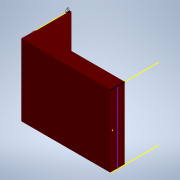
# Autodesk Inventor part: LPS_base
Saved by Autodesk Inventor 2022 (Build 260153000, 153)
## iProperties
Created: 2024-07-06
Part Number: LPS_base
Material: Типовые
Document SubType Name: Modeling
Designer: Капустяник Андрей
Density: 1 g/cm^3
Appearance: По умолчанию
Author: Капустяник Андрей
Autodesk Inventor part; units mm, degrees
ref_plane "YZ Plane" through (0, 0, 0) normal (1, 0, 0) x (0, 1, 0)
ref_plane "XZ Plane" through (0, 0, 0) normal (0, 1, 0) x (-1, 0, 0)
ref_plane "XY Plane" through (0, 0, 0) normal (0, 0, 1) x (1, 0, 0)
sketch "Эскиз1" plane through (0, 0, 0) normal (0, 0, 1) x (1, 0, 0)
  line L0 (29.9444, -74.6554) -> (-27.0756, -74.6554) projected
  line L1 (29.9444, 31.7946) -> (29.9444, -74.6554) projected
  line L2 (-27.0756, 31.7946) -> (29.9444, 31.7946) projected
  line L3 (-27.0756, -74.6554) -> (-27.0756, 31.7946) projected
  circle A0 centre (-22.2656, 27.6646) radius 2 projected
  circle A1 centre (-22.2656, -70.5254) radius 2 projected
  circle A2 centre (25.1344, -70.5254) radius 2 projected
  circle A3 centre (25.1344, 27.6646) radius 2 projected
  line L4 (-29.0756, 55) -> (29.0756, 55)
  line L5 (29.0756, 55) -> (29.0756, -55)
  line L6 (29.0756, -55) -> (-29.0756, -55)
  line L7 (-29.0756, -55) -> (-29.0756, 55)
  line L8 (-29.0756, 55) -> (29.0756, -55) construction
  line L9 (29.0756, 55) -> (-29.0756, -55) construction
  line L10 (-32.0756, 58) -> (32.0756, 58)
  line L11 (32.0756, 58) -> (32.0756, -58)
  line L12 (32.0756, -58) -> (-32.0756, -58)
  line L13 (-32.0756, -58) -> (-32.0756, 58)
  line L14 (29.0756, 55) -> (109.0756, 55)
  line L15 (109.0756, 55) -> (109.0756, -55)
  line L16 (109.0756, -55) -> (29.0756, -55)
  line L17 (32.0756, -58) -> (112.0756, -58)
  line L18 (112.0756, -58) -> (112.0756, 58)
  line L19 (112.0756, 58) -> (32.0756, 58)
  point P0 (0, 0)
  dimension "d0" = 110
  dimension "d1" = 2
  dimension "d2" = 3
  dimension "d3" = 80
  dimension "d4" = 80
  constraints: 32 end point, 6 parallel, 6 perpendicular, 2 midpoint, 1 horizontal, 3 other
  measures "d0" distance of L4.end L5.end
  measures "d1" distance between parallel lines of L3 L7
  measures "d2" distance between parallel lines of L7 L13
  measures "d3" distance of L4.end L14.end
  measures "d4" distance of L11.end L17.end
extrude "Выдавливание1" add sketch "Эскиз1" along normal blind 3 contours L12 L3 L6 L16 L1 | L1 L16 L11 L12 | L12 L13 L10 L11 L14 L4 L7 L6 L3 | L16 L5 L2 L1 | L1 L2 L5 L14 L11 L16 | L11 L16 L15 L14 L19 L18 L17 | L6 L7 L4 L5 L2 L3 | L3 L2 L5 L6 | L11 L14 L15 L16 | A0 | A3
sketch "Эскиз2" plane through (0, 0, 0) normal (0, 0, -1) x (-1, 0, 0)
  line L0 (-112.0756, -58) -> (-112.0756, 58) projected
  line L1 (32.0756, -58) -> (-112.0756, -58) projected
  line L2 (32.0756, 58) -> (32.0756, -58) projected
  line L3 (-112.0756, 58) -> (32.0756, 58) projected
  line L4 (-109.0756, -55) -> (-109.0756, 55)
  line L5 (-109.0756, 55) -> (29.0756, 55)
  line L6 (29.0756, 55) -> (29.0756, -55)
  line L7 (29.0756, -55) -> (-109.0756, -55)
  point P0 (0, 0)
  dimension "d7" = 3
  constraints: 8 end point, 3 other
  measures "d7" distance between parallel lines of L1 L7
extrude "Выдавливание2" add sketch "Эскиз2" along normal blind 75
sketch "Эскиз3" plane through (-32.0756, 58, 3) normal (0, 1, 0) x (1, 0, 0)
  line L0 (3, 3) -> (3, 78) projected
  line L1 (3, 78) -> (78, 3)
  line L2 (3, 3) -> (141.1512, 3) projected
  line L3 (0, 78) -> (0, 0) projected
  line L4 (144.1512, 0) -> (0, 0) projected
  line L5 (144.1512, 78) -> (144.1512, 0) projected
  line L6 (0, 78) -> (144.1512, 78) projected
  line L7 (141.1512, 3) -> (141.1512, 78) projected
  line L8 (141.1512, 3) -> (144.1512, 3)
  line L9 (144.1512, 78) -> (144.1512, 0) projected
  line L10 (144.1512, 3) -> (144.1512, 18)
  line L11 (144.1512, 0) -> (144.1512, 78) projected
  line L12 (144.1512, 18) -> (63, 18)
  line L13 (135.5856, 23) -> (56.5656, 23) projected
  line L14 (58, 23) -> (144.1512, 23)
  point P0 (32.0756, 3)
  point P1 (78, 3)
  point P2 (3, 78)
  point P3 (144.1512, 3)
  point P4 (144.1512, 18)
  point P5 (58, 23)
  point P6 (134.1512, 23)
  dimension "d10" = 45
  dimension "d13" = 15
  constraints: 8 end point, 6 point on line, 1 horizontal, 1 perpendicular, 6 other
  measures "d13" distance of L8.end L10.end
extrude "Выдавливание3" cut sketch "Эскиз3" against normal up to surface (116 mm away) contours L6 L7 L14 L13 L1 | L6 L5 L14 L7
sketch "Эскиз4" plane through (-32.0756, -58, 3) normal (-1, 0, 0) x (0, 0, 1)
  line L0 (-78, 116) -> (-78, 113) projected
  line L1 (-78, 116) -> (-72, 116)
  line L2 (-23, 116) -> (-78, 116) projected
  line L3 (-72, 116) -> (-72, 0)
  line L4 (-78, 0) -> (0, 0) projected
  point P0 (-3, 58)
  point P1 (-18, 116)
  point P2 (-3, 116)
  dimension "d14" = 6
  constraints: 4 end point, 2 point on line, 1 perpendicular
  measures "d14" distance of L0.start L1.end
sketch "Эскиз5" plane through (112.0756, -58, 3) normal (1, 0, 0) x (0, 0, -1)
  line L0 (78, 116) -> (0, 116) projected
  line L1 (23, 116) -> (0, 116)
  line L2 (11.5, 116) -> (11.5, 0)
  line L3 (78, 0) -> (0, 0) projected
  point P0 (3, 58)
  constraints: 4 end point, 2 point on line, 1 collinear, 1 midpoint, 1 vertical
